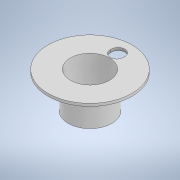
# Autodesk Inventor part: O-Ring
Saved by Autodesk Inventor 2022 (Build 260153000, 153)
## iProperties
Created: 2022-02-10
Part Number: O-Ring
Material: Generic
Document SubType Name: Modeling
Designer: Vedic
Density: 1 g/cm^3
Appearance: Default
Author: Vedic
Autodesk Inventor part; units mm, degrees
ref_plane "YZ Plane" through (0, 0, 0) normal (1, 0, 0) x (0, 1, 0)
ref_plane "XZ Plane" through (0, 0, 0) normal (0, 1, 0) x (-1, 0, 0)
ref_plane "XY Plane" through (0, 0, 0) normal (0, 0, 1) x (1, 0, 0)
sketch "Sketch1" plane through (0, 0, 0) normal (0, 1, 0) x (-1, 0, 0)
  circle A0 centre (0, 0) radius 16.5
  circle A1 centre (0, 0) radius 14.75
  dimension "d0" = 33
  dimension "d1" = 29.5
  constraints: 2 centre point, 2 coincident
  measures "d0" diameter of A0
  measures "d1" diameter of A1
extrude "Extrusion1" add sketch "Sketch1" along normal blind 25.4
sketch "Sketch2" plane through (0, 25.4, 0) normal (0, 1, 0) x (1, 0, 0)
  circle A0 centre (0, 0) radius 14.75
  circle A1 centre (0, 0) radius 31.75
  circle A2 centre (0, 0) radius 14.75 projected
  dimension "d5" = 63.5
  dimension "d6" = 0
  constraints: 2 centre point, 2 coincident
  measures "d5" diameter of A1
  measures "d6" radial gap between concentric circles of A2 A0
extrude "Extrusion2" add sketch "Sketch2" along normal blind 2
sketch "Sketch3" plane through (0, 25.4, 0) normal (0, -1, 0) x (1, 0, 0)
  circle A0 centre (0, -20.32) radius 5
  circle A1 centre (0, -21.32) radius 5
  line L0 (0, -20.32) -> (0, -21.32)
  line L1 (5, -20.32) -> (5, -21.32)
  line L2 (-5, -20.32) -> (-5, -21.32)
  point P0 (0, 0)
  point P1 (4.9749, -20.82)
  point P2 (-4.9749, -20.82)
  dimension "d9" = 10
  dimension "d10" = 1
  dimension "d11" = 20.32
  constraints: 6 end point, 4 point on circle, 2 centre point, 2 vertical, 1 equal radius, 1 parallel, 1 tangent
  measures "d9" diameter of A0
  measures "d10" distance of L0.start L0.end
  measures "d11" distance of point (0, 0) L0.start
extrude "Extrusion3" cut sketch "Sketch3" against normal blind 2 contours A0 A1 | A1 A0 | A0 A1
body "Solid1"
